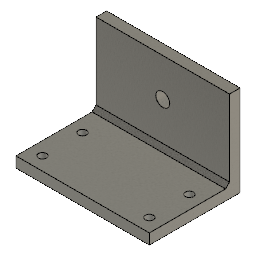
Base del motor v1 (Autodesk Fusion 360 design; units mm, degrees)
Autodesk Fusion 360 part; units mm, degrees
sketch "Boceto1" plane through (0, 0, 0) normal (0, 0, 1) x (1, 0, 0)
  line L0 (50, -34) -> (-50, -34)
  line L1 (-50, -34) -> (-50, 34)
  line L2 (-50, 34) -> (50, 34)
  line L3 (50, 34) -> (50, -34)
  line L4 (50, -34) -> (-50, 34) construction
  line L5 (-50, -34) -> (50, 34) construction
  circle A0 centre (-40, 6) radius 3
  circle A1 centre (-40, -24) radius 3
  line L6 (0, -34) -> (0, 34) construction
  circle A2 centre (40, 6) radius 3
  circle A3 centre (40, -24) radius 3
  dimension "d1" = 100
  dimension "d2" = 68
  dimension "d3" = 6
  dimension "d4" = 6
  dimension "d5" = 30
  dimension "d6" = 10
  dimension "d7" = 10
  dimension "d8" = 10
  constraint horizontal L0
  constraint perpendicular L0 L1
  constraint parallel L0 L2
  constraint parallel L1 L3
  constraint coincident L4 origin
  constraint coincident L5 origin
  constraint midpoint L0 L6.start
  constraint midpoint L2 L6.end
  constraint symmetric A0 L6 A2
  constraint symmetric A1 L6 A3
  measures "d1" distance of L0.start L0.end
  measures "d2" distance of L0.start L2.end
  measures "d3" diameter of A0
  measures "d4" diameter of A1
  measures "d5" vertical distance of A0.centre A1.centre
  measures "d6" distance of L1 A1.centre
  measures "d7" distance of L1 A0.centre
  measures "d8" distance of L0 A1.centre
extrude "Extruir1" add sketch "Boceto1" along normal blind 8
sketch "Boceto2" plane through (0, 34, 0) normal (0, 1, 0) x (-1, 0, 0)
  line L0 (-50, 0) -> (50, 0)
  line L1 (50, 0) -> (50, 8)
  line L2 (50, 8) -> (-50, 8)
  line L3 (-50, 8) -> (-50, 0)
  line L4 (-50, 0) -> (-50, 68)
  line L5 (-50, 68) -> (50, 68)
  line L6 (50, 68) -> (50, 0)
  circle A0 centre (0, 39.5) radius 5.175
  dimension "d16" = 68
  dimension "d17" = 10.35
  dimension "d18" = 50
  dimension "d19" = 28.5
  constraint coincident L0.start L3.end
  constraint perpendicular L0 L4
  constraint perpendicular L4 L5
  constraint coincident L0.end L1.start
  constraint perpendicular L0 L6
  measures "d16" distance of L0.start L4.end
  measures "d17" diameter of A0
  measures "d18" distance of L4 A0.centre
  measures "d19" distance of L5 A0.centre
extrude "Extruir2" add sketch "Boceto2" against normal blind 8 contours L2 L4 L5 L6
chamfer "Chaflán1" distance 3 angle 45 1 edges at (0, 26, 8)
